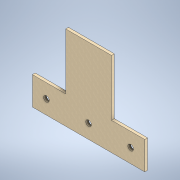
# Autodesk Inventor part: aussenOben
Saved by Autodesk Inventor 2020.3 (Build 243373010, 373A)
## iProperties
Created: 2021-02-11
Part Number: aussenOben
Material: Generisch
Document SubType Name: Modeling
Designer: Stefan
Density: 1 g/cm^3
Appearance: Pappel
Author: Stefan
Autodesk Inventor part; units mm, degrees
ref_plane "YZ Plane" through (0, 0, 0) normal (1, 0, 0) x (0, 1, 0)
ref_plane "XZ Plane" through (0, 0, 0) normal (0, 1, 0) x (-1, 0, 0)
ref_plane "XY Plane" through (0, 0, 0) normal (0, 0, 1) x (1, 0, 0)
sketch "Skizze1" plane through (0, 0, 0) normal (0, 0, 1) x (1, 0, 0)
  line L0 (163.1081, -200) -> (163.1081, 0)
  line L1 (163.1081, 0) -> (0, 0)
  line L2 (0, 0) -> (0, -200)
  line L3 (0, -200) -> (-118.4459, -200)
  line L4 (-118.4459, -200) -> (-118.4459, -300)
  line L5 (-118.4459, -300) -> (281.5541, -300)
  line L6 (281.5541, -300) -> (281.5541, -200)
  line L7 (281.5541, -200) -> (163.1081, -200)
  circle A0 centre (231.5541, -250) radius 10
  circle A1 centre (-68.4459, -250) radius 10
  circle A2 centre (81.5541, -250) radius 10
  dimension "d0" = 20
  dimension "d1" = 90
  dimension "d2" = 118.4459
  dimension "d3" = 281.5541
  dimension "d4" = 400
  dimension "d5" = 200
  dimension "d6" = 100
  dimension "d7" = 281.5541
  dimension "d8" = 200
  dimension "d9" = 200
  dimension "d10" = 0
  dimension "d11" = 0
  dimension "d12" = 100
  dimension "d13" = 0
  dimension "d14" = 50
  dimension "d15" = 50
  dimension "d16" = 200
  dimension "d17" = 118.4459
  dimension "d18" = 0
  dimension "d19" = 118.4459
  dimension "d20" = 200
  dimension "d21" = 50
  dimension "d22" = 200
  dimension "d23" = 281.5541
  dimension "d24" = 0
  dimension "d25" = 281.5541
  dimension "d26" = 350
  dimension "d27" = 50
  dimension "d28" = 0
  dimension "d29" = 400
  dimension "d30" = 100
  dimension "d31" = 400
  constraints: 16 end point, 5 parallel, 3 centre point, 2 equal radius, 1 horizontal, 1 vertical
  measures "d0" diameter of A0
  measures "d1" angle of L6 L3
  measures "d2" distance between parallel lines of L0 L6
  measures "d3" distance between parallel lines of L2 L6
  measures "d4" distance between parallel lines of L4 L6
  measures "d5" distance between parallel lines of L1 L7
  measures "d6" distance between parallel lines of L5 L7
  measures "d7" distance from line of point (0, 0) L6
  measures "d8" distance from line of point (0, 0) L7
  measures "d9" distance from line of point (0, 0) L3
  measures "d10" distance from line of L6.end L7
  measures "d11" distance from line of L7.start L6
  measures "d12" distance from line of L6.start L7
  measures "d13" distance from line of L5.end L6
  measures "d14" distance from line of A0.centre L6
  measures "d15" distance from line of A0.centre L7
  measures "d16" distance from line of L0.end L7
  measures "d17" distance from line of L1.start L6
  measures "d18" distance from line of L0.start L7
  measures "d19" distance from line of L7.end L6
  measures "d20" distance from line of A2.centre L6
  measures "d21" distance from line of A2.centre L7
  measures "d22" distance from line of L2.start L7
  measures "d23" distance from line of L1.end L6
  measures "d24" distance from line of L2.end L7
  measures "d25" distance from line of L3.start L6
  measures "d26" distance from line of A1.centre L6
  measures "d27" distance from line of A1.centre L7
  measures "d28" distance from line of L4.start L7
  measures "d29" distance from line of L3.end L6
  measures "d30" distance from line of L4.end L7
  measures "d31" distance from line of L5.start L6
extrude "Extrusion1" add sketch "Skizze1" along normal blind 10
